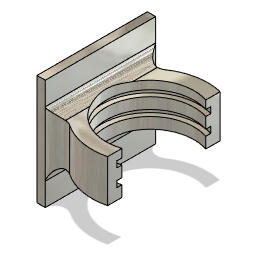
Pump Holder v2 (Autodesk Fusion 360 design; units mm, degrees)
Autodesk Fusion 360 part; units mm, degrees
sketch "Sketch1" plane through (0, 0, 0) normal (0, 1, 0) x (1, 0, 0)
  circle A0 centre (0, 0) radius 16
  circle A1 centre (0, 0) radius 21
  dimension "d1" = 32
  dimension "d2" = 42
  constraint coincident A0.centre A1.centre
  measures "d1" diameter of A0
  measures "d2" diameter of A1
extrude "Extrude1" add sketch "Sketch1" along normal blind 4
sketch "Sketch2" plane through (0, 4, 0) normal (0, 1, 0) x (-1, 0, 0)
  circle A0 centre (0, 0) radius 16
  circle A1 centre (0, 0) radius 21
  circle A2 centre (0, 0) radius 17.75
  circle A3 centre (0, 0) radius 21
  dimension "d5" = 35.5
  dimension "d6" = 42
  constraint coincident A0.centre A1.centre
  constraint concentric A2 A3
  measures "d5" diameter of A2
  measures "d6" diameter of A3
extrude "Extrude2" add sketch "Sketch2" along normal blind 2.2 contours A1 A3
sketch "Sketch3" plane through (0, 6.2, 0) normal (0, 1, 0) x (-1, 0, 0)
  circle A0 centre (0, 0) radius 17.75
  circle A1 centre (0, 0) radius 21
  circle A2 centre (0, 0) radius 16
  circle A3 centre (0, 0) radius 21
  dimension "d9" = 32
  dimension "d10" = 42
  constraint concentric A0 A2
  constraint coincident A0.centre A1.centre
  measures "d9" diameter of A2
  measures "d10" diameter of A3
extrude "Extrude3" add sketch "Sketch3" along normal blind 4 contours A0 | A1 A3
sketch "Sketch4" plane through (0, 10.2, 0) normal (0, 1, 0) x (-1, 0, 0)
  circle A0 centre (0, 0) radius 16
  circle A1 centre (0, 0) radius 21
  circle A2 centre (0, 0) radius 17.75
  circle A3 centre (0, 0) radius 21
  dimension "d13" = 35.5
  constraint coincident A0.centre A1.centre
  constraint concentric A2 A3
  measures "d13" diameter of A2
extrude "Extrude4" add sketch "Sketch4" along normal blind 2.2 contours A1 A3
sketch "Sketch5" plane through (0, 12.4, 0) normal (0, 1, 0) x (-1, 0, 0)
  circle A0 centre (0, 0) radius 17.75
  circle A1 centre (0, 0) radius 21
  circle A2 centre (0, 0) radius 16
  circle A3 centre (0, 0) radius 21
  dimension "d16" = 32
  dimension "d17" = 42
  constraint concentric A0 A2
  constraint concentric A2 A3
  measures "d16" diameter of A2
  measures "d17" diameter of A3
extrude "Extrude5" add sketch "Sketch5" along normal blind 3 contours A0 | A1 A3
sketch "Sketch6" plane through (0, 15.4, 0) normal (0, 1, 0) x (-1, 0, 0)
  circle A0 centre (0, 0) radius 16
  circle A1 centre (0, 0) radius 21
  line L0 (-25, -25) -> (-5, -25)
  line L1 (-5, -25) -> (-5, 25)
  line L2 (-5, 25) -> (-25, 25)
  line L3 (-25, 25) -> (-25, -25)
  dimension "d20" = 50
  dimension "d21" = 25
  dimension "d22" = 25
  dimension "d23" = 5
  constraint horizontal L0
  constraint vertical L1
  constraint horizontal L2
  constraint vertical L3
  measures "d20" distance of L0 L2
  measures "d21" distance of A0.centre L0
  measures "d22" distance of A0.centre L3
  measures "d23" distance of A0.centre L1
extrude "Extrude6" cut sketch "Sketch6" against normal up to surface (15.4 mm away) contours A0 L1 | A0 A1 L1 | A1 L0 L1 L2 L3 picked at (-8.6522, -0.3927) picked at (-19.2425, 1.4237)
ref_plane "WorkPlane1" through (-18, 7.7, -17.7974) normal (1, 0, 0) x (0, 0, 1)
sketch "Sketch7" plane through (-18, 7.7, -17.7974) normal (1, 0, 0) x (0, 0, -1)
  line L0 (2.5987, 7.7) -> (2.5987, -7.7)
  line L1 (3.2026, -7.7) -> (-38.7974, -7.7)
  line L2 (-38.1935, -7.7) -> (-38.1935, 7.7)
  line L3 (3.2026, 7.7) -> (-38.7974, 7.7)
  line L4 (2.2026, 20) -> (-37.7974, 20)
  line L5 (-37.7974, 20) -> (-37.7974, -20)
  line L6 (-37.7974, -20) -> (2.2026, -20)
  line L7 (2.2026, -20) -> (2.2026, 20)
  dimension "d27" = 40
  dimension "d28" = 40
  dimension "d29" = 1
  dimension "d30" = 20
  constraint horizontal L4
  constraint vertical L5
  constraint horizontal L6
  constraint vertical L7
  measures "d27" distance of L4.start L4.end
  measures "d28" distance of L4.start L6.end
  measures "d29" distance of L3.end L5
  measures "d30" distance of origin L4
extrude "Extrude7" add sketch "Sketch7" against normal blind 3 contours L1 L3 L5 L7 | L3 L4 L5 L7 | L1 L5 L6 L7
fillet "Fillet1" radius 4 2 edges at (-18, 7.7, 10.8167) (-18, 7.7, -10.8167)
fillet "Fillet2" radius 4 2 edges at (-18, 15.4, 0) (-18, 0, 0)
